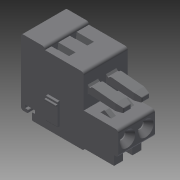
# Autodesk Inventor part: 734-102
Saved by Autodesk Inventor 2014 (Build 180170000, 170)
## iProperties
Category: Control System
Company: Autodesk Inc.
Created: 2013-12-21
Part Number: 734-102
Description: Power connector 2 pole
Document SubType Name: Modeling
Designer: Autodesk Inc.
Density: 1 g/cm^3
Vendor: Wago
Catalog Web Link: http://www.wagocatalog.com/okv3/index.asp?cid=51&lid=5&str_from_home=first
Material: Generic
Appearance: Light Gray
Title: 734-102
Author: Autodesk Inc.
Autodesk Inventor part; units mm, degrees
ref_plane "YZ Plane" through (0, 0, 0) normal (1, 0, 0) x (0, 1, 0)
ref_plane "XZ Plane" through (0, 0, 0) normal (0, 1, 0) x (-1, 0, 0)
ref_plane "XY Plane" through (0, 0, 0) normal (0, 0, 1) x (1, 0, 0)
sketch "Skizze_1" plane through (0, 0, 0) normal (0, 0, 1) x (1, 0, 0)
  arc A0 (0, 1.3) -> (0.5, 0.8) centre (0.5, 1.3) ccw
  line L0 (0.5, 0.8) -> (1.2, 0.8)
  arc A1 (1.2, 0.8) -> (1.4, 1) centre (1.2, 1) ccw
  line L1 (1.4, 1) -> (1.4, 1.2)
  arc A2 (1.4, 1.2) -> (1.2, 1.4) centre (1.2, 1.2) ccw
  line L2 (1.2, 1.4) -> (0.9, 1.4)
  arc A3 (0.8, 1.5) -> (0.9, 1.4) centre (0.9, 1.5) ccw
  line L3 (0.8, 1.5) -> (0.8, 1.9)
  arc A4 (0.9, 2) -> (0.8, 1.9) centre (0.9, 1.9) ccw
  line L4 (0.9, 2) -> (2.6, 2)
  arc A5 (2.7, 1.9) -> (2.6, 2) centre (2.6, 1.9) ccw
  line L5 (2.7, 1.9) -> (2.7, 1.5)
  arc A6 (2.6, 1.4) -> (2.7, 1.5) centre (2.6, 1.5) ccw
  line L6 (2.6, 1.4) -> (2.3, 1.4)
  arc A7 (2.3, 1.4) -> (2.1, 1.2) centre (2.3, 1.2) ccw
  line L7 (2.1, 1.2) -> (2.1, 0.2)
  arc A8 (2.1, 0.2) -> (2.3, 0) centre (2.3, 0.2) ccw
  line L8 (2.3, 0) -> (11.8, 0)
  arc A9 (11.8, 0) -> (12, 0.2) centre (11.8, 0.2) ccw
  line L9 (12, 0.2) -> (12, 2.1)
  line L10 (12, 2.1) -> (18.1, 2.1)
  arc A10 (18.1, 2.1) -> (18.6, 2.6) centre (18.1, 2.6) ccw
  line L11 (18.6, 2.6) -> (18.6, 6.1)
  arc A11 (18.6, 6.1) -> (18.1, 6.6) centre (18.1, 6.1) ccw
  line L12 (18.1, 6.6) -> (12, 6.6)
  line L13 (12, 6.6) -> (12, 12.4)
  arc A12 (12, 12.4) -> (11.5, 12.9) centre (11.5, 12.4) ccw
  line L14 (11.5, 12.9) -> (4.6, 12.9)
  line L15 (4.6, 12.9) -> (4.6, 12.91)
  arc A13 (4.6, 12.91) -> (4.11, 13.4) centre (4.11, 12.91) ccw
  line L16 (4.11, 13.4) -> (0.5, 13.4)
  arc A14 (0.5, 13.4) -> (0, 12.9) centre (0.5, 12.9) ccw
  line L17 (0, 12.9) -> (0, 1.3)
  constraints: 36 end point, 30 point on circle, 15 centre point
extrude "Extrusion1" add sketch "Skizze_1" along normal blind 7
sketch "Skizze_3" plane through (0, 0, 0) normal (0, 0, 1) x (1, 0, 0)
  circle A0 centre (1.5, 12.2) radius 0.9
  constraints: 1 centre point
extrude "Extrusion2" add sketch "Skizze_3" against normal blind 1.5
sketch "Skizze_4" plane through (0, 0, 0) normal (0, 0, 1) x (1, 0, 0)
  circle A0 centre (3.4, 12.2) radius 0.9
  constraints: 1 centre point
extrude "Extrusion3" add sketch "Skizze_4" against normal blind 1.5
sketch "Skizze_5" plane through (0, 0, 0) normal (0, 0, 1) x (1, 0, 0)
  circle A0 centre (8.9, 11.7) radius 0.89
  constraints: 1 centre point
extrude "Extrusion4" add sketch "Skizze_5" against normal blind 1.5
sketch "Skizze_6" plane through (0, 0, 0) normal (0, 0, 1) x (1, 0, 0)
  circle A0 centre (10.7, 11.7) radius 0.89
  constraints: 1 centre point
extrude "Extrusion5" add sketch "Skizze_6" against normal blind 1.5
sketch "Skizze_7" plane through (0, 0, 0) normal (0, 0, 1) x (1, 0, 0)
  circle A0 centre (4.3, 1.4) radius 1
  constraints: 1 centre point
extrude "Extrusion6" add sketch "Skizze_7" against normal blind 1.5
sketch "Skizze_8" plane through (0, 0, 0) normal (0, 0, 1) x (1, 0, 0)
  circle A0 centre (7.6, 1.4) radius 1
  constraints: 1 centre point
extrude "Extrusion7" add sketch "Skizze_8" against normal blind 1.5
sketch "Skizze_9" plane through (0, 0, 0) normal (0, 0, 1) x (1, 0, 0)
  circle A0 centre (10.7, 1.4) radius 1
  constraints: 1 centre point
extrude "Extrusion8" add sketch "Skizze_9" against normal blind 1.5
sketch "Skizze_2" plane through (0, 0, 0) normal (0, 0, 1) x (1, 0, 0)
  arc A0 (0, 2.6) -> (0.5, 2.1) centre (0.5, 2.6) ccw
  line L0 (0.5, 2.1) -> (2.6, 2.1)
  arc A1 (2.8, 1.9) -> (2.6, 2.1) centre (2.6, 1.9) ccw
  line L1 (2.8, 1.9) -> (2.8, 1.5)
  arc A2 (2.6, 1.3) -> (2.8, 1.5) centre (2.6, 1.5) ccw
  line L2 (2.6, 1.3) -> (2.3, 1.3)
  arc A3 (2.3, 1.3) -> (2.2, 1.2) centre (2.3, 1.2) ccw
  line L3 (2.2, 1.2) -> (2.2, 0.2)
  arc A4 (2.2, 0.2) -> (2.4, 0) centre (2.4, 0.2) ccw
  line L4 (2.4, 0) -> (11.5, 0)
  arc A5 (11.5, 0) -> (12, 0.5) centre (11.5, 0.5) ccw
  line L5 (12, 0.5) -> (12, 12.4)
  arc A6 (12, 12.4) -> (11.5, 12.9) centre (11.5, 12.4) ccw
  line L6 (11.5, 12.9) -> (4.6, 12.9)
  line L7 (4.6, 12.9) -> (4.6, 12.91)
  arc A7 (4.6, 12.91) -> (4.11, 13.4) centre (4.11, 12.91) ccw
  line L8 (4.11, 13.4) -> (0.5, 13.4)
  arc A8 (0.5, 13.4) -> (0, 12.9) centre (0.5, 12.9) ccw
  line L9 (0, 12.9) -> (0, 2.6)
  constraints: 20 end point, 18 point on circle, 9 centre point
extrude "Extrusion9" add sketch "Skizze_2" against normal blind 1.4
sketch "Skizze_10" plane through (0, 4.35, 0) normal (0, 1, 0) x (1, 0, 0)
  line L0 (18.6, -1.75) -> (17.3, -1.75)
  line L1 (17.3, -1.75) -> (17.3, -1)
  line L2 (17.3, -1) -> (17.5, -1)
  line L3 (17.5, -1) -> (18.6, -0.25)
  line L4 (18.6, -0.25) -> (18.6, -1.75)
  line L5 (18.6, -1.75) -> (17.3, -1.75)
  constraints: 12 end point
revolve "Revolution1" cut sketch "Skizze_10" angle 360 about axis through (18.6, 4.35, 1.75) along (1, 0, 0)
pattern_linear "Rectangular Pattern1" count 2 spacing 3.5 along (0, 0, 1) of "Revolution1"
sketch "Skizze_12" plane through (4.6, 0, 0) normal (1, 0, 0) x (0, 0, -1)
  line L0 (-5.75, 12.9) -> (-5.6, 11.8)
  line L1 (-5.6, 11.8) -> (-4.6, 11.8)
  line L2 (-4.6, 11.8) -> (-4.45, 12.9)
  line L3 (-4.45, 12.9) -> (-5.75, 12.9)
  constraints: 8 end point
extrude "Extrusion10" cut sketch "Skizze_12" along normal blind 3.3
pattern_linear "Rectangular Pattern2" count 2 spacing 3.5 along (0, 0, -1) of "Extrusion10"
sketch "Skizze_14" plane through (0, 0, 0) normal (1, 0, 0) x (0, 1, 0)
  line L0 (11.2, 6.4) -> (8.3, 6.4)
  line L1 (8.3, 6.4) -> (8.3, 3.5)
  line L2 (8.3, 3.5) -> (11.2, 3.5)
  line L3 (11.2, 3.5) -> (11.2, 6.4)
  constraints: 8 end point
extrude "Extrusion11" cut sketch "Skizze_14" along normal blind 1
pattern_linear "Rectangular Pattern3" count 2 spacing 3.5 along (0, 0, -1) of "Extrusion11"
sketch "Skizze_16" plane through (0, 0, 0) normal (1, 0, 0) x (0, 1, 0)
  arc A0 (3, 6.7) -> (2.5, 6.2) centre (3, 6.2) ccw
  line L0 (2.5, 6.2) -> (2.5, 4)
  arc A1 (2.5, 4) -> (3, 3.5) centre (3, 4) ccw
  line L1 (3, 3.5) -> (6.3, 3.5)
  arc A2 (6.3, 3.5) -> (6.5, 3.7) centre (6.3, 3.7) ccw
  line L2 (6.5, 3.7) -> (6.5, 4.1)
  line L3 (6.5, 4.1) -> (6.9, 4.1)
  arc A3 (6.9, 4.1) -> (6.9, 6.1) centre (6.9, 5.1) ccw
  line L4 (6.9, 6.1) -> (6.5, 6.1)
  line L5 (6.5, 6.1) -> (6.5, 6.5)
  arc A4 (6.5, 6.5) -> (6.3, 6.7) centre (6.3, 6.5) ccw
  line L6 (6.3, 6.7) -> (3, 6.7)
  constraints: 14 end point, 10 point on circle, 5 centre point
extrude "Extrusion12" cut sketch "Skizze_16" along normal blind 1
pattern_linear "Rectangular Pattern4" count 2 spacing 3.5 along (0, 0, -1) of "Extrusion12"
sketch "Skizze_18" plane through (0, 0, 1.75) normal (0, 0, 1) x (1, 0, 0)
  line L0 (13.9, 6.6) -> (15.9489, 6.6)
  line L1 (15.9489, 6.6) -> (14.7828, 7.2732)
  arc A0 (14.7828, 7.2732) -> (14.5414, 7.2414) centre (14.6828, 7.1) ccw
  line L2 (14.5414, 7.2414) -> (13.9, 6.6)
  constraints: 6 end point, 2 point on circle, 1 centre point
extrude "Extrusion13" add sketch "Skizze_18" along normal mid plane 0.9
sketch "Skizze_19" plane through (0, 0, 5.25) normal (0, 0, 1) x (1, 0, 0)
  line L0 (13.9, 6.6) -> (15.9489, 6.6)
  line L1 (15.9489, 6.6) -> (14.7828, 7.2732)
  arc A0 (14.7828, 7.2732) -> (14.5414, 7.2414) centre (14.6828, 7.1) ccw
  line L2 (14.5414, 7.2414) -> (13.9, 6.6)
  constraints: 6 end point, 2 point on circle, 1 centre point
extrude "Extrusion14" add sketch "Skizze_19" along normal mid plane 0.9
sketch "Skizze_20" plane through (0, 0, 1.8) normal (0, 0, 1) x (1, 0, 0)
  line L0 (12, 0.35) -> (17.8, 0.35)
  line L1 (17.8, 0.35) -> (17.8, 2.35)
  line L2 (17.8, 2.35) -> (12, 2.35)
  line L3 (12, 2.35) -> (12, 0.35)
  constraints: 8 end point
extrude "Extrusion15" add sketch "Skizze_20" along normal blind 1.7
sketch "Skizze_21" plane through (0, 0, 5.3) normal (0, 0, 1) x (1, 0, 0)
  line L0 (12, 0.35) -> (17.8, 0.35)
  line L1 (17.8, 0.35) -> (17.8, 2.35)
  line L2 (17.8, 2.35) -> (12, 2.35)
  line L3 (12, 2.35) -> (12, 0.35)
  constraints: 8 end point
extrude "Extrusion16" add sketch "Skizze_21" along normal blind 1.7
sketch "Skizze_22" plane through (0, 0, 5.25) normal (0, 0, 1) x (1, 0, 0)
  arc A0 (12.2113, 9.088) -> (12, 8.8884) centre (12.2, 8.8884) ccw
  line L0 (12.2113, 9.088) -> (17.3, 8.8)
  line L1 (17.3, 8.8) -> (18.4174, 8.8978)
  arc A1 (18.4174, 8.8978) -> (18.6, 9.097) centre (18.4, 9.097) ccw
  line L2 (18.6, 9.097) -> (18.6, 9.5982)
  arc A2 (18.6, 9.5982) -> (18.4518, 9.7914) centre (18.4, 9.5982) ccw
  line L3 (18.4518, 9.7914) -> (17.3, 10.1)
  line L4 (17.3, 10.1) -> (13.0466, 10.4978)
  arc A3 (13.0466, 10.4978) -> (12.5417, 10.2) centre (13, 10) ccw
  line L5 (12.5417, 10.2) -> (12.3, 10.2)
  line L6 (12.3, 10.2) -> (12, 10.5)
  line L7 (12, 10.5) -> (12, 8.8884)
  constraints: 16 end point, 8 point on circle, 4 centre point
extrude "Extrusion17" add sketch "Skizze_22" along normal mid plane 2
pattern_linear "Rectangular Pattern5" count 2 spacing 3.5 along (0, 0, -1) of "Extrusion17"
sketch "Skizze_24" plane through (0, 8.6, 0) normal (0, 1, 0) x (1, 0, 0)
  line L0 (17.3, -3.05) -> (18.9, -3.05)
  line L1 (18.9, -3.05) -> (18.9, -0.45)
  line L2 (18.9, -0.45) -> (17.3, -0.45)
  line L3 (17.3, -0.45) -> (17.3, -0.75)
  line L4 (17.3, -0.75) -> (18.4435, -1.0048)
  arc A0 (18.6, -1.2) -> (18.4435, -1.0048) centre (18.4, -1.2) ccw
  line L5 (18.6, -1.2) -> (18.6, -2.3)
  arc A1 (18.4435, -2.4952) -> (18.6, -2.3) centre (18.4, -2.3) ccw
  line L6 (18.4435, -2.4952) -> (17.3, -2.75)
  line L7 (17.3, -2.75) -> (17.3, -3.05)
  constraints: 16 end point, 4 point on circle, 2 centre point
extrude "Extrusion18" cut sketch "Skizze_24" along normal blind 1.7
pattern_linear "Rectangular Pattern6" count 2 spacing 3.5 along (0, 0, 1) of "Extrusion18"
sketch "Skizze_26" plane through (7.4, 0, 0) normal (1, 0, 0) x (0, 0, -1)
  arc A0 (-7.7, 5.3) -> (-7.6, 5.2) centre (-7.6, 5.3) ccw
  line L0 (-7.6, 5.2) -> (-7.4, 5.2)
  line L1 (-7.4, 5.2) -> (-7.4, 1.8)
  arc A1 (-7.4, 1.8) -> (-7.3, 1.7) centre (-7.3, 1.8) ccw
  line L2 (-7.3, 1.7) -> (-7, 1.7)
  line L3 (-7, 1.7) -> (-7, 5.9)
  line L4 (-7, 5.9) -> (-7.3, 5.9)
  arc A2 (-7.3, 5.9) -> (-7.4, 5.8) centre (-7.3, 5.8) ccw
  line L5 (-7.4, 5.8) -> (-7.4, 5.5)
  line L6 (-7.4, 5.5) -> (-7.6, 5.5)
  arc A3 (-7.6, 5.5) -> (-7.7, 5.4) centre (-7.6, 5.4) ccw
  line L7 (-7.7, 5.4) -> (-7.7, 5.3)
  constraints: 16 end point, 8 point on circle, 4 centre point
extrude "Extrusion19" add sketch "Skizze_26" against normal blind 2.2
body "Solid1"
